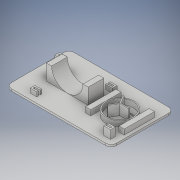
# Autodesk Inventor part: base
Saved by Autodesk Inventor 2019 (Build 230136000, 136)
## iProperties
Created: 2022-02-03
Part Number: base
Material: Generic
Document SubType Name: Modeling
Designer: josec
Density: 1 g/cm^3
Appearance: Default
Author: josec
Autodesk Inventor part; units mm, degrees
ref_plane "YZ Plane" through (0, 0, 0) normal (1, 0, 0) x (0, 1, 0)
ref_plane "XZ Plane" through (0, 0, 0) normal (0, 1, 0) x (-1, 0, 0)
ref_plane "XY Plane" through (0, 0, 0) normal (0, 0, 1) x (1, 0, 0)
sketch "Sketch1" plane through (0, 0, 0) normal (0, 1, 0) x (-1, 0, 0)
  line L0 (0, 0) -> (-90, 0)
  line L1 (-90, 0) -> (-90, -60)
  line L2 (-90, -60) -> (0, -60)
  line L3 (0, -60) -> (0, 0)
  dimension "d0" = 90
  dimension "d1" = 60
  constraints: 8 end point, 2 parallel, 1 horizontal, 1 perpendicular
  measures "d0" distance of L2.end L1.end
  measures "d1" distance of L1.end L0.end
extrude "Extrusion1" add sketch "Sketch1" along normal blind 2
sketch "Sketch2" plane through (0, 2, 0) normal (0, 1, 0) x (1, 0, 0)
  line L0 (90, 0) -> (90, 60) construction
  line L1 (90, 60) -> (77.25, 60) construction
  line L2 (90, 60) -> (0, 60) construction
  line L3 (77.25, 60) -> (77.25, 0) construction
  line L4 (0, 0) -> (90, 0) construction
  line L5 (77.25, 30) -> (77.25, 35.5) construction
  line L6 (77.25, 35.5) -> (77.25, 30) construction
  line L7 (77.25, 30) -> (77.25, 24.5) construction
  line L8 (77.25, 24.5) -> (71.25, 24.5)
  line L9 (71.25, 24.5) -> (71.25, 23.5)
  line L10 (71.25, 23.5) -> (77.25, 23.5)
  line L11 (77.25, 23.5) -> (77.25, 24.5)
  line L12 (77.25, 35.5) -> (71.25, 35.5)
  line L13 (71.25, 35.5) -> (71.25, 36.5)
  line L14 (71.25, 36.5) -> (77.25, 36.5)
  line L15 (77.25, 36.5) -> (77.25, 35.5)
  dimension "d4" = 12.75
  dimension "d5" = 5.5
  dimension "d6" = 5.5
  dimension "d7" = 6
  dimension "d8" = 1
  dimension "d9" = 1
  constraints: 26 end point, 4 parallel, 4 point on line, 2 horizontal, 2 perpendicular, 1 collinear, 1 midpoint, 1 vertical
  measures "d4" distance of L0.end L1.end
  measures "d5" distance of L5.start L5.end
  measures "d6" distance of L5.start L7.end
  measures "d7" distance of L10.end L9.end
  measures "d8" distance of L9.end L8.end
  measures "d9" distance of L12.end L13.end
extrude "Extrusion2" cut sketch "Sketch2" against normal through all
sketch "Sketch3" plane through (0, 2, 0) normal (0, 1, 0) x (1, 0, 0)
  line L0 (77.25, 35.5) -> (71.25, 35.5) construction
  line L1 (77.25, 24.5) -> (71.25, 24.5) construction
  line L2 (71.25, 35.5) -> (71.25, 24.5) construction
  line L3 (71.25, 30) -> (64.75, 30) construction
  line L4 (64.75, 30) -> (64.75, 32.5) construction
  line L5 (64.75, 32.5) -> (59.75, 32.5) construction
  line L6 (59.75, 32.5) -> (59.75, 27.5) construction
  line L7 (59.75, 27.5) -> (64.75, 27.5) construction
  line L8 (64.75, 27.5) -> (64.75, 32.5) construction
  line L9 (59.75, 27.5) -> (62.75, 27.5) construction
  line L10 (59.75, 32.5) -> (62.75, 32.5) construction
  arc A0 (62.75, 27.5) -> (62.75, 32.5) centre (62.1875, 30) ccw
  line L11 (62.75, 32.5) -> (59.75, 32.5) construction
  line L12 (59.75, 32.5) -> (59.75, 27.5) construction
  line L13 (59.75, 32.5) -> (62.75, 32.5)
  line L14 (59.75, 32.5) -> (59.75, 27.5)
  line L15 (59.75, 27.5) -> (62.75, 27.5)
  point P0 (0, 0)
  dimension "d12" = 6.5
  dimension "d15" = 2.5
  dimension "d16" = 5
  dimension "d17" = 5
  dimension "d18" = 3
  dimension "d19" = 3
  constraints: 28 end point, 4 perpendicular, 3 point on circle, 2 collinear, 2 horizontal, 2 parallel, 2 point on line, 2 vertical, 1 centre point, 1 midpoint
  measures "d12" distance of L3.start L3.end
  measures "d15" distance of L3.end L4.end
  measures "d16" distance of L7.end L6.end
  measures "d17" distance of L6.end L5.end
  measures "d18" distance of L6.end L9.end
  measures "d19" distance of L5.end L10.end
extrude "Extrusion3" cut sketch "Sketch3" against normal through all
sketch "Sketch20" plane through (0, 2, 0) normal (0, 1, 0) x (1, 0, 0)
  line L0 (77.25, 36.5) -> (77.25, 35.5) construction
  line L1 (77.25, 36.5) -> (59.75, 36.5) construction
  line L2 (59.75, 23.5) -> (77.25, 23.5) construction
  line L3 (77.25, 23.5) -> (77.25, 36.5) construction
  line L4 (68.5, 30) -> (77.25, 30) construction
  line L5 (68.5, 30) -> (68.5, 29.5) construction
  line L6 (68.5, 29.5) -> (77.25, 29.5)
  line L7 (77.25, 29.5) -> (77.25, 30.5)
  line L8 (77.25, 30.5) -> (68.5, 30.5)
  line L9 (68.5, 30.5) -> (68.5, 29.5)
  line L10 (68.933, 30.25) -> (64.558, 37.8277)
  line L11 (63.692, 37.3277) -> (68.067, 29.75)
  line L12 (68.067, 29.75) -> (68.933, 30.25)
  line L13 (69.7542, 40.8277) -> (58.4958, 34.3277) construction
  line L14 (68.067, 30.25) -> (63.692, 22.6723)
  line L15 (64.558, 22.1723) -> (68.933, 29.75)
  line L16 (68.933, 29.75) -> (68.067, 30.25)
  line L17 (58.4958, 25.6723) -> (69.7542, 19.1723) construction
  line L18 (63.692, 37.3277) -> (64.558, 37.8277)
  line L19 (63.692, 22.6723) -> (64.558, 22.1723)
  point P0 (0, 0)
  point P1 (64.125, 37.5777)
  point P2 (64.125, 22.4223)
  dimension "d143" = 13
  dimension "d144" = 0.5
  dimension "d145" = 1
  dimension "d148" = 360
  constraints: 38 end point, 3 parallel, 3 point on line, 2 collinear, 2 horizontal, 2 perpendicular, 1 midpoint, 34 other
  measures "d143" distance of L2.start L1.end
  measures "d144" distance of L4.start L5.end
  measures "d145" distance of L7.end L6.end
extrude "Extrusion17" add sketch "Sketch20" along normal blind 10
sketch "Sketch21" plane through (0, 2, 0) normal (0, 1, 0) x (1, 0, 0)
  line L0 (77.25, 24.5) -> (77.25, 23.5) construction
  line L1 (77.25, 23.5) -> (59.75, 23.5) construction
  line L2 (59.75, 23.5) -> (59.75, 36.5) construction
  line L3 (59.75, 36.5) -> (77.25, 36.5) construction
  line L4 (77.25, 36.5) -> (77.25, 23.5) construction
  circle A0 centre (68.5, 30) radius 12.5
  circle A1 centre (68.5, 30) radius 13.5
  point P0 (0, 0)
  dimension "d154" = 13
  dimension "d155" = 25
  dimension "d156" = 27
  constraints: 8 end point, 2 centre point, 2 parallel, 1 coincident, 1 horizontal, 1 perpendicular
  measures "d154" distance of L1.end L2.end
  measures "d155" diameter of A0
  measures "d156" diameter of A1
extrude "Extrusion18" add sketch "Sketch21" along normal blind 5
sketch "Sketch23" plane through (0, 2, 0) normal (0, 1, 0) x (1, 0, 0)
  line L0 (90, 0) -> (90, 60) construction
  line L1 (90, 30) -> (87, 30) construction
  line L2 (87, 30) -> (87, 18.5) construction
  line L3 (87, 18.5) -> (50, 18.5) construction
  line L4 (50, 18.5) -> (50, 41.5) construction
  line L5 (50, 41.5) -> (87, 41.5) construction
  line L6 (87, 41.5) -> (87, 18.5) construction
  line L7 (87, 18.5) -> (87, 15.5) construction
  line L8 (87, 15.5) -> (82, 15.5) construction
  line L9 (87, 15.5) -> (82, 15.5)
  line L10 (82, 15.5) -> (82, 44.5)
  line L11 (82, 44.5) -> (87, 44.5)
  line L12 (87, 44.5) -> (87, 15.5)
  line L13 (50, 18.5) -> (50, 15.5) construction
  line L14 (50, 15.5) -> (55, 15.5)
  line L15 (55, 15.5) -> (55, 44.5)
  line L16 (55, 44.5) -> (50, 44.5)
  line L17 (50, 44.5) -> (50, 15.5)
  point P0 (0, 0)
  dimension "d164" = 3
  dimension "d165" = 11.5
  dimension "d166" = 37
  dimension "d167" = 23
  dimension "d168" = 3
  dimension "d169" = 5
  dimension "d170" = 5
  dimension "d171" = 29
  dimension "d172" = 3
  dimension "d173" = 5
  dimension "d174" = 29
  constraints: 34 end point, 6 parallel, 4 horizontal, 4 perpendicular, 3 vertical, 1 midpoint
  measures "d164" distance of L1.start L1.end
  measures "d165" distance of L1.end L2.end
  measures "d166" distance of L4.end L5.end
  measures "d167" distance of L3.end L4.end
  measures "d168" distance of L2.end L7.end
  measures "d169" distance of L7.end L8.end
  measures "d170" distance of L10.end L11.end
  measures "d171" distance of L9.end L10.end
  measures "d172" distance of L3.end L13.end
  measures "d173" distance of L16.end L15.end
  measures "d174" distance of L15.end L14.end
extrude "Extrusion19" add sketch "Sketch23" along normal blind 5
sketch "Sketch24" plane through (0, 2, 0) normal (0, 1, 0) x (1, 0, 0)
  line L0 (84, 8.5) -> (82.5, 8.5) construction
  line L1 (82.5, 8.5) -> (8.5, 8.5) construction
  line L2 (8.5, 8.5) -> (8.5, 6.9) construction
  line L3 (8.5, 6.9) -> (82.5, 6.9) construction
  line L4 (82.5, 6.9) -> (82.5, 8.5) construction
  line L5 (82.5, 6.9) -> (77.5, 6.9)
  line L6 (77.5, 6.9) -> (77.5, 5.4)
  line L7 (77.5, 5.4) -> (84, 5.4)
  line L8 (82.5, 6.9) -> (82.5, 8.5)
  line L9 (82.5, 8.5) -> (77.5, 8.5)
  line L10 (77.5, 8.5) -> (77.5, 10)
  line L11 (8.5, 6.9) -> (13.5, 6.9)
  line L12 (13.5, 6.9) -> (13.5, 5.4)
  line L13 (13.5, 5.4) -> (7, 5.4)
  line L14 (8.5, 8.5) -> (13.5, 8.5)
  line L15 (13.5, 8.5) -> (13.5, 10)
  line L16 (13.5, 10) -> (7, 10)
  line L17 (7, 10) -> (7, 5.4)
  line L18 (8.5, 6.9) -> (8.5, 8.5)
  line L19 (77.5, 10) -> (84, 10)
  line L20 (84, 5.4) -> (84, 10)
  line L21 (84, 8.5) -> (90, 8.5) construction
  line L22 (90, 0) -> (90, 60) construction
  line L23 (87, 44.5) -> (87, 15.5) construction
  line L24 (87, 15.5) -> (90, 15.5) construction
  line L25 (90, 8.5) -> (90, 15.5) construction
  point P0 (0, 0)
  dimension "d178" = 1.5
  dimension "d179" = 74
  dimension "d180" = 1.6
  dimension "d181" = 5
  dimension "d182" = 1.5
  dimension "d183" = 5
  dimension "d184" = 1.5
  dimension "d185" = 5
  dimension "d186" = 1.5
  dimension "d187" = 6.5
  dimension "d188" = 5
  dimension "d189" = 1.5
  dimension "d230" = 6
  dimension "d231" = 7
  constraints: 48 end point, 9 perpendicular, 6 point on line, 4 horizontal, 2 parallel, 2 vertical, 1 collinear
  measures "d178" distance of L0.start L0.end
  measures "d179" distance of L3.end L2.end
  measures "d180" distance of L2.end L1.end
  measures "d181" distance of L3.end L5.end
  measures "d182" distance of L5.end L6.end
  measures "d183" distance of L0.end L9.end
  measures "d184" distance of L9.end L10.end
  measures "d185" distance of L2.end L11.end
  measures "d186" distance of L11.end L12.end
  measures "d187" distance of L12.end L13.end
  measures "d188" distance of L1.end L14.end
  measures "d189" distance of L14.end L15.end
  measures "d230" distance of L0.start L21.end
  measures "d231" distance between parallel lines of L21 L24
extrude "Extrusion20" add sketch "Sketch24" along normal blind 4
sketch "Sketch25" plane through (0, 6, 0) normal (0, 1, 0) x (1, 0, 0)
  line L0 (84, 5.4) -> (84, 10) projected
  line L1 (77.5, 5.4) -> (84, 5.4)
  line L2 (84, 5.4) -> (84, 10)
  line L3 (84, 10) -> (77.5, 10) projected
  line L4 (84, 10) -> (77.5, 10)
  line L5 (77.5, 10) -> (77.5, 8.5) projected
  line L6 (77.5, 10) -> (77.5, 8.5)
  line L7 (77.5, 8.5) -> (82.5, 8.5) projected
  line L8 (77.5, 8.5) -> (82.5, 8.5)
  line L9 (82.5, 6.9) -> (82.5, 8.5) projected
  line L10 (82.5, 8.5) -> (82.5, 6.9)
  line L11 (82.5, 6.9) -> (77.5, 6.9)
  line L12 (77.5, 5.4) -> (77.5, 6.9)
  point P0 (0, 0)
  constraints: 16 end point, 4 perpendicular, 2 collinear, 1 horizontal, 1 vertical
extrude "Extrusion21" add sketch "Sketch25" along normal blind 4
sketch "Sketch26" plane through (0, 2, 0) normal (0, 1, 0) x (1, 0, 0)
  line L0 (50, 15.5) -> (55, 15.5) projected
  line L1 (45, 23) -> (5, 23)
  line L2 (5, 23) -> (5, 38)
  line L3 (5, 38) -> (45, 38)
  line L4 (45, 38) -> (45, 23)
  line L5 (50, 15.5) -> (50, 0) construction
  line L6 (50, 0) -> (45, 0) construction
  line L7 (0, 0) -> (90, 0) construction
  line L8 (45, 23) -> (45, 0) construction
  dimension "d195" = 40
  dimension "d196" = 15
  dimension "d229" = 23
  constraints: 14 end point, 2 parallel, 2 perpendicular, 1 horizontal, 1 midpoint, 1 vertical
  measures "d195" distance of L2.end L3.end
  measures "d196" distance of L1.end L2.end
  measures "d229" distance of L1.start L6.end
extrude "Extrusion22" add sketch "Sketch26" along normal blind 15
sketch "Sketch27" plane through (45, 2, -38) normal (0, 0, -1) x (-1, 0, 0)
  line L0 (40, 15) -> (0, 15) projected
  circle A0 centre (20, 15) radius 15
  point P0 (45, -2)
  dimension "d199" = 30
  constraints: 1 centre point, 1 midpoint
  measures "d199" diameter of A0
extrude "Extrusion23" cut sketch "Sketch27" against normal blind 15
sketch "Sketch29" plane through (0, 2, 0) normal (0, 1, 0) x (1, 0, 0)
  line L0 (25, 38) -> (45, 38) projected
  line L1 (45, 38) -> (45, 46) construction
  line L2 (45, 46) -> (-7, 46) construction
  line L3 (-7, 46) -> (-7, 47.6) construction
  line L4 (-7, 47.6) -> (45, 47.6) construction
  line L5 (45, 47.6) -> (45, 46) construction
  line L6 (45, 46) -> (40, 46)
  line L7 (40, 46) -> (40, 44.5)
  line L8 (40, 44.5) -> (46.5, 44.5)
  line L9 (45, 46) -> (45, 47.6)
  line L10 (45, 47.6) -> (40, 47.6)
  line L11 (40, 47.6) -> (40, 49.1)
  line L12 (40, 49.1) -> (46.5, 49.1)
  line L13 (46.5, 49.1) -> (46.5, 44.5)
  line L14 (-7, 47.6) -> (-7, 46)
  line L15 (-7, 46) -> (-2, 46)
  line L16 (-2, 46) -> (-2, 44.5)
  line L17 (-2, 44.5) -> (-8.5, 44.5)
  line L18 (-7, 47.6) -> (-2, 47.6)
  line L19 (-2, 47.6) -> (-2, 49.1)
  line L20 (-2, 49.1) -> (-8.5, 49.1)
  line L21 (-8.5, 49.1) -> (-8.5, 44.5)
  point P0 (0, 0)
  dimension "d215" = 8
  dimension "d216" = 52
  dimension "d217" = 1.6
  dimension "d218" = 5
  dimension "d219" = 1.5
  dimension "d220" = 6.5
  dimension "d221" = 1.5
  dimension "d222" = 5
  dimension "d223" = 6.5
  dimension "d224" = 6.5
  constraints: 42 end point, 7 perpendicular, 5 vertical, 4 point on line, 2 horizontal, 2 parallel, 1 collinear
  measures "d215" distance of L0.end L1.end
  measures "d216" distance of L3.end L4.end
  measures "d217" distance of L2.end L3.end
  measures "d218" distance of L1.end L6.end
  measures "d219" distance of L6.end L7.end
  measures "d220" distance of L7.end L8.end
  measures "d221" distance of L10.end L11.end
  measures "d222" distance of L2.end L15.end
  measures "d223" distance of L16.end L17.end
  measures "d224" distance of L19.end L20.end
extrude "Extrusion25" add sketch "Sketch29" along normal blind 4
sketch "Sketch30" plane through (0, 0, -60) normal (-1, 0, 0) x (0, 0, 1)
  line L0 (0, 0) -> (0, 2) projected
  line L1 (60, 0) -> (60, 2) projected
  line L2 (0, 0) -> (60, 0)
  line L3 (60, 0) -> (60, 2)
  line L4 (60, 2) -> (0, 2)
  line L5 (0, 2) -> (0, 0)
  constraints: 8 end point, 2 parallel, 1 horizontal, 1 perpendicular
extrude "Extrusion26" add sketch "Sketch30" along normal blind 10.5
sketch "Sketch31" plane through (0, 2, 0) normal (0, 1, 0) x (1, 0, 0)
  arc A0 (90, 55) -> (85, 60) centre (85, 55) ccw
  arc A1 (-10.5, 5) -> (-5.5, 0) centre (-5.5, 5) ccw
  arc A2 (-5.5, 60) -> (-10.5, 55) centre (-5.5, 55) ccw
  arc A3 (85, 0) -> (90, 5) centre (85, 5) ccw
  line L0 (90, 0) -> (85, 0)
  line L1 (90, 0) -> (90, 5)
  line L2 (-5.5, 0) -> (-10.5, 0)
  line L3 (-10.5, 55) -> (-10.5, 60)
  line L4 (-10.5, 60) -> (-5.5, 60)
  line L5 (85, 60) -> (90, 60)
  line L6 (90, 60) -> (90, 55)
  line L7 (-10.5, 0) -> (-10.5, 5)
  point P0 (0, 0)
  dimension "d232" = 5
  constraints: 16 end point, 8 point on circle, 4 centre point, 3 equal radius, 2 perpendicular, 2 tangent, 1 horizontal, 1 vertical
  measures "d232" radius of A0
extrude "Extrusion27" cut sketch "Sketch31" against normal through all
body "Solid1"
